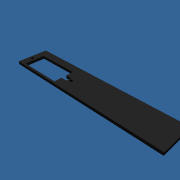
# Autodesk Inventor part: Acrylic_UpperArm_Support
Saved by Autodesk Inventor 2012 (Build 160160000, 160)
## iProperties
Created: 2014-03-29
Part Number: Acrylic_UpperArm_Support
Material: Default
Document SubType Name: Modeling
Designer: Admin
Density: 1 g/cm^3
Author: Admin
Autodesk Inventor part; units mm, degrees
ref_plane "YZ Plane" through (0, 0, 0) normal (1, 0, 0) x (0, 1, 0)
ref_plane "XZ Plane" through (0, 0, 0) normal (0, 1, 0) x (-1, 0, 0)
ref_plane "XY Plane" through (0, 0, 0) normal (0, 0, 1) x (1, 0, 0)
sketch "Sketch1" plane through (0, 0, 0) normal (0, 0, 1) x (1, 0, 0)
  line L0 (-30, -15) -> (-30, 15)
  line L1 (-30, 15) -> (120, 15)
  line L2 (120, 15) -> (120, -15)
  line L3 (120, -15) -> (-30, -15)
  line L4 (-60, 0) -> (150, 0) projected
  line L5 (0, -21) -> (0, 21) projected
  dimension "d13" = 30
  dimension "d55" = 150
  dimension "d56" = 15
  constraints: 8 end point, 1 horizontal, 1 parallel, 1 perpendicular
  measures "d13" distance of L1.end L2.end
  measures "d55" distance of L2.end L0.start
  measures "d56" distance between parallel lines of L1 L4
extrude "Extrusion1" add sketch "Sketch1" along normal blind 2.8
sketch "Sketch4" plane through (0, 0, 2.8) normal (0, 0, 1) x (1, 0, 0)
  line L0 (-60, 0) -> (150, 0) projected
  line L1 (17.9, 9.9) -> (17.9, 2.5)
  line L2 (-22.4, 9.9) -> (17.9, 9.9)
  line L3 (17.9, 2.5) -> (23.9, 2.5)
  line L4 (23.9, 2.5) -> (23.9, -2.5)
  line L5 (23.9, -2.5) -> (17.9, -2.5)
  line L6 (17.9, -2.5) -> (17.9, -9.9)
  line L7 (17.9, -9.9) -> (-22.4, -9.9)
  line L8 (-22.4, -9.9) -> (-22.4, 9.9)
  line L9 (-22.4, 9.9) -> (17.9, 9.9)
  circle A0 centre (26.7, 0) radius 1.5
  circle A1 centre (-26.2, 0) radius 1.5
  line L10 (120, 15) -> (120, -15) projected
  line L11 (120, -15) -> (-30, -15) projected
  line L12 (112.8, 2.5) -> (115, 2.5)
  line L13 (115, 2.5) -> (115, -2.5)
  line L14 (115, -2.5) -> (112.8, -2.5)
  line L15 (112.8, -2.5) -> (112.8, 2.5)
  line L16 (97.8, 2.5) -> (100, 2.5)
  line L17 (100, 2.5) -> (100, -2.5)
  line L18 (100, -2.5) -> (97.8, -2.5)
  line L19 (97.8, -2.5) -> (97.8, 2.5)
  line L20 (82.8, 2.5) -> (85, 2.5)
  line L21 (85, 2.5) -> (85, -2.5)
  line L22 (85, -2.5) -> (82.8, -2.5)
  line L23 (82.8, -2.5) -> (82.8, 2.5)
  line L24 (67.8, 2.5) -> (70, 2.5)
  line L25 (70, 2.5) -> (70, -2.5)
  line L26 (70, -2.5) -> (67.8, -2.5)
  line L27 (67.8, -2.5) -> (67.8, 2.5)
  line L28 (52.8, 2.5) -> (55, 2.5)
  line L29 (55, 2.5) -> (55, -2.5)
  line L30 (55, -2.5) -> (52.8, -2.5)
  line L31 (52.8, -2.5) -> (52.8, 2.5)
  line L32 (37.8, 2.5) -> (40, 2.5)
  line L33 (40, 2.5) -> (40, -2.5)
  line L34 (40, -2.5) -> (37.8, -2.5)
  line L35 (37.8, -2.5) -> (37.8, 2.5)
  line L36 (112.8, -7.5) -> (115, -7.5)
  line L37 (115, -7.5) -> (115, -12.5)
  line L38 (115, -12.5) -> (112.8, -12.5)
  line L39 (112.8, -12.5) -> (112.8, -7.5)
  line L40 (97.8, -7.5) -> (100, -7.5)
  line L41 (100, -7.5) -> (100, -12.5)
  line L42 (100, -12.5) -> (97.8, -12.5)
  line L43 (97.8, -12.5) -> (97.8, -7.5)
  line L44 (82.8, -7.5) -> (85, -7.5)
  line L45 (85, -7.5) -> (85, -12.5)
  line L46 (85, -12.5) -> (82.8, -12.5)
  line L47 (82.8, -12.5) -> (82.8, -7.5)
  line L48 (67.8, -7.5) -> (70, -7.5)
  line L49 (70, -7.5) -> (70, -12.5)
  line L50 (70, -12.5) -> (67.8, -12.5)
  line L51 (67.8, -12.5) -> (67.8, -7.5)
  line L52 (52.8, -7.5) -> (55, -7.5)
  line L53 (55, -7.5) -> (55, -12.5)
  line L54 (55, -12.5) -> (52.8, -12.5)
  line L55 (52.8, -12.5) -> (52.8, -7.5)
  line L56 (37.8, -7.5) -> (40, -7.5)
  line L57 (40, -7.5) -> (40, -12.5)
  line L58 (40, -12.5) -> (37.8, -12.5)
  line L59 (37.8, -12.5) -> (37.8, -7.5)
  line L60 (112.8, 12.5) -> (112.8, 7.5)
  line L61 (115, 12.5) -> (112.8, 12.5)
  line L62 (112.8, 7.5) -> (115, 7.5)
  line L63 (115, 7.5) -> (115, 12.5)
  line L64 (97.8, 12.5) -> (97.8, 7.5)
  line L65 (100, 12.5) -> (97.8, 12.5)
  line L66 (97.8, 7.5) -> (100, 7.5)
  line L67 (100, 7.5) -> (100, 12.5)
  line L68 (82.8, 12.5) -> (82.8, 7.5)
  line L69 (85, 12.5) -> (82.8, 12.5)
  line L70 (82.8, 7.5) -> (85, 7.5)
  line L71 (85, 7.5) -> (85, 12.5)
  line L72 (67.8, 12.5) -> (67.8, 7.5)
  line L73 (70, 12.5) -> (67.8, 12.5)
  line L74 (67.8, 7.5) -> (70, 7.5)
  line L75 (70, 7.5) -> (70, 12.5)
  line L76 (52.8, 12.5) -> (52.8, 7.5)
  line L77 (55, 12.5) -> (52.8, 12.5)
  line L78 (52.8, 7.5) -> (55, 7.5)
  line L79 (55, 7.5) -> (55, 12.5)
  line L80 (37.8, 12.5) -> (37.8, 7.5)
  line L81 (40, 12.5) -> (37.8, 12.5)
  line L82 (37.8, 7.5) -> (40, 7.5)
  line L83 (40, 7.5) -> (40, 12.5)
  circle A2 centre (106.4, 0) radius 1.5
  circle A3 centre (91.4, 0) radius 1.5
  circle A4 centre (76.4, 0) radius 1.5
  circle A5 centre (61.4, 0) radius 1.5
  circle A6 centre (46.4, 0) radius 1.5
  dimension "d57" = 2.2
  dimension "d58" = 5
  dimension "d59" = 2.5
  dimension "d60" = 5
  dimension "d63" = 15
  dimension "d66" = 10
  dimension "d69" = 3
  dimension "d70" = 6.4
  dimension "d73" = 15
  constraints: 162 end point, 24 symmetric about line, 8 horizontal, 7 centre point, 5 vertical, 2 parallel, 1 perpendicular, 1 point on line, 108 other
  measures "d57" distance of L13.end L14.end
  measures "d58" distance of L12.end L13.end
  measures "d59" distance between parallel lines of L0 L12
  measures "d60" distance between parallel lines of L10 L13
  measures "d63" distance of L12.start L19.end
  measures "d66" distance of L12.start L39.end
  measures "d69" diameter of A2
  measures "d70" distance from line of L15 A2.centre
  measures "d73" distance of A2.centre A3.centre
extrude "Extrusion3" cut sketch "Sketch4" against normal through all
equation "\"d56\" = 0.5 * d13"
body "Solid1"
